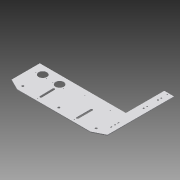
# Autodesk Inventor part: Side-Wall
Saved by Autodesk Inventor 2014 (Build 180170000, 170)
## iProperties
Created: 2013-09-08
Part Number: Side-Wall
Material: Generic
Document SubType Name: Sheet Metal
Designer: hensgen3
Density: 1 g/cm^3
Sheet Metal Rule: Default
Appearance: Aluminum - Polished
Author: hensgen3
Autodesk Inventor part; units mm, degrees
ref_plane "YZ Plane" through (0, 0, 0) normal (1, 0, 0) x (0, 1, 0)
ref_plane "XZ Plane" through (0, 0, 0) normal (0, 1, 0) x (-1, 0, 0)
ref_plane "XY Plane" through (0, 0, 0) normal (0, 0, 1) x (1, 0, 0)
sketch "Sketch1" plane through (0, 0, 0) normal (0, 1, 0) x (-1, 0, 0)
  line L0 (-236.5637, 132.8889) -> (195.2363, 132.8889)
  line L1 (195.2363, 132.8889) -> (195.2363, -19.5111)
  line L2 (195.2363, -19.5111) -> (-236.5637, -19.5111)
  line L3 (-236.5637, -19.5111) -> (-236.5637, 132.8889)
  point P0 (0, 0)
  dimension "d0" = 431.8
  dimension "d2" = 152.4
  measures "d0" distance of L0.start L0.end
  measures "d2" distance of L2.end L0.start
extrude "Plate1" add sketch "Sketch1" along normal blind 3.175
sketch "Sketch2" plane through (0, 3.175, 0) normal (0, 1, 0) x (1, 0, 0)
  line L0 (-195.2363, -132.8889) -> (-195.2363, 19.5111) projected
  line L1 (236.5637, -132.8889) -> (-195.2363, -132.8889) projected
  line L2 (236.5637, 19.5111) -> (236.5637, -132.8889) projected
  line L3 (-195.2363, 19.5111) -> (236.5637, 19.5111) projected
  circle A0 centre (-144.4363, -107.4889) radius 50.8
  line L4 (20.6637, -132.8889) -> (20.6637, -82.0889)
  line L5 (185.7637, -132.8889) -> (185.7637, -82.0889)
  line L6 (-144.4363, -107.4889) -> (-144.4363, -132.8889)
  line L7 (-144.4363, -107.4889) -> (-195.2363, -107.4889)
  line L8 (20.6637, -107.4889) -> (20.6637, -110.6639)
  circle A1 centre (20.6637, -110.6639) radius 50.8
  circle A2 centre (185.7637, -107.4889) radius 50.8
  circle A3 centre (-144.4363, -107.4889) radius 4.7625
  line L9 (-144.4363, -56.6889) -> (185.7637, -56.6889)
  line L10 (-144.4363, -158.2889) -> (185.7637, -158.2889)
  circle A4 centre (20.6637, -110.6639) radius 4.7625
  circle A5 centre (185.7637, -107.4889) radius 4.7625
  point P0 (0, 0)
  dimension "d13" = 50.8
  dimension "d14" = 25.4
  dimension "d15" = 50.8
  dimension "d16" = 3.175
  dimension "d17" = 101.6
  dimension "d18" = 101.6
  dimension "d19" = 9.525
  dimension "d20" = 50.8
  dimension "d21" = 9.525
  dimension "d22" = 9.525
  constraints: 14 end point, 6 centre point, 5 point on circle, 4 coincident, 4 point on line, 3 midpoint, 3 perpendicular, 2 tangent, 1 parallel
  measures "d13" distance of L6.start L7.end
  measures "d14" distance of L6.start L6.end
  measures "d15" distance of L0.start L6.end
  measures "d16" distance of L8.start L8.end
  measures "d17" diameter of A1
  measures "d18" diameter of A2
  measures "d19" diameter of A3
  measures "d20" distance from line of L2 L5.end
  measures "d21" diameter of A4
  measures "d22" diameter of A5
extrude "Cut1" cut sketch "Sketch2" against normal blind 3.175 contours A3 L6 L7 | L7 L6 A3 | L4 A4 | L4 A4 | A5 L5 | L5 A5
sketch "Sketch3" plane through (0, 3.175, 0) normal (0, 1, 0) x (1, 0, 0)
  circle A0 centre (-144.4363, -107.4889) radius 4.7625 projected
  circle A1 centre (20.6637, -110.6639) radius 4.7625 projected
  circle A2 centre (185.7637, -107.4889) radius 4.7625 projected
  line L0 (-195.2363, -132.8889) -> (-195.2363, 19.5111) projected
  line L1 (236.5637, -132.8889) -> (-195.2363, -132.8889) projected
  line L2 (236.5637, 19.5111) -> (236.5637, -132.8889) projected
  circle A3 centre (-144.4363, -107.4889) radius 50.8
  circle A4 centre (20.6637, -110.6639) radius 50.8
  circle A5 centre (185.7637, -107.4889) radius 50.8
  line L3 (-195.2363, -107.4889) -> (-144.4363, -132.8889)
  line L4 (236.5637, -107.4889) -> (185.7637, -132.8889)
  point P0 (0, 0)
  dimension "d25" = 101.6
  dimension "d27" = 101.6
  dimension "d26" = 101.6
  dimension "d31" = 50.8
  dimension "d32" = 50.8
  constraints: 4 end point, 4 point on line, 3 coincident, 2 horizontal alignment, 1 centre point, 4 other
  measures "d26" diameter of A4
  measures "d31" horizontal distance of L3.start L3.end
  measures "d32" horizontal distance of L4.start L4.end
extrude "Cut2" cut sketch "Sketch3" against normal blind 3.175 contours L0 A3 L1 | L3 L1 A3 | L1 A5 L2 | L1 L4 A5 picked at (-178.0457, -118.896) picked at (219.3731, -118.896)
sketch "Sketch4" plane through (0, 3.175, 0) normal (0, 1, 0) x (1, 0, 0)
  line L0 (185.7637, -132.8889) -> (236.5637, -107.4889) projected
  line L1 (236.5637, 19.5111) -> (236.5637, -107.4889) projected
  line L2 (-195.2363, 19.5111) -> (236.5637, 19.5111) projected
  line L3 (-195.2363, -107.4889) -> (-195.2363, 19.5111) projected
  line L4 (-195.2363, -107.4889) -> (-144.4363, -132.8889) projected
  line L5 (185.7637, -132.8889) -> (-144.4363, -132.8889) projected
  circle A0 centre (185.7637, -107.4889) radius 4.7625 projected
  circle A1 centre (20.6637, -110.6639) radius 4.7625 projected
  circle A2 centre (-144.4363, -107.4889) radius 4.7625 projected
  circle A3 centre (-144.4363, -107.4889) radius 50.8
  circle A4 centre (20.6637, -110.6639) radius 50.8
  circle A5 centre (185.7637, -107.4889) radius 50.8
  point P0 (0, 0)
  dimension "d35" = 101.6
  dimension "d36" = 101.6
  dimension "d37" = 101.6
  constraints: 3 centre point, 3 coincident
  measures "d35" diameter of A3
  measures "d36" diameter of A4
  measures "d37" diameter of A5
sketch "Sketch5" plane through (0, 3.175, 0) normal (0, 1, 0) x (1, 0, 0)
  line L0 (185.7637, -132.8889) -> (236.5637, -107.4889) projected
  line L1 (236.5637, 19.5111) -> (236.5637, -107.4889) projected
  line L2 (-195.2363, 19.5111) -> (236.5637, 19.5111) projected
  line L3 (-195.2363, -107.4889) -> (-195.2363, 19.5111) projected
  line L4 (-195.2363, -107.4889) -> (-144.4363, -132.8889) projected
  line L5 (185.7637, -132.8889) -> (-144.4363, -132.8889) projected
  circle A0 centre (185.7637, -107.4889) radius 4.7625 projected
  circle A1 centre (20.6637, -110.6639) radius 4.7625 projected
  circle A2 centre (-144.4363, -107.4889) radius 4.7625 projected
  point P0 (0, 0)
sketch "Sketch6" plane through (0, 3.175, 0) normal (0, 1, 0) x (1, 0, 0)
  line L0 (-195.2363, 19.5111) -> (236.5637, 19.5111) projected
  circle A0 centre (-144.4363, -107.4889) radius 4.7625 projected
  line L1 (-144.4363, -107.4889) -> (-144.4363, 19.5111)
  circle A1 centre (-144.4363, -17.9889) radius 37.5
  circle A2 centre (-68.2363, -17.9889) radius 19.05
  circle A3 centre (-144.4363, -17.9889) radius 18.7706
  circle A4 centre (-68.2363, -17.9889) radius 18.7706
  point P0 (0, 0)
  dimension "d39" = 75
  dimension "d40" = 38.1
  dimension "d41" = 76.2
  dimension "d42" = 37.5412
  dimension "d43" = 37.5412
  constraints: 4 centre point, 2 end point, 2 point on line, 1 coincident, 1 perpendicular, 1 tangent
  measures "d39" diameter of A1
  measures "d40" diameter of A2
  measures "d41" distance of A2.centre A1.centre
  measures "d42" diameter of A3
  measures "d43" diameter of A4
extrude "Cut3" cut sketch "Sketch6" against normal blind 3.175 contours A3 L1 | L1 A3 | A4
sketch "Sketch7" plane through (0, 3.175, 0) normal (0, 1, 0) x (1, 0, 0)
  arc A0 (-36.2323, -12.4614) -> (-39.4073, -9.2864) centre (-39.4073, -12.4614) ccw
  line L0 (-39.4073, -9.2864) -> (-42.3918, -9.2864)
  line L1 (-42.3918, -9.2864) -> (-42.3918, -15.2554)
  line L2 (-42.3918, -15.2554) -> (-49.6689, -15.2554)
  arc A1 (-86.8037, -15.2554) -> (-49.6689, -15.2554) centre (-68.2363, -17.9889) ccw
  line L3 (-86.8037, -15.2554) -> (-94.0808, -15.2554)
  line L4 (-94.0808, -15.2554) -> (-94.0808, -9.2864)
  line L5 (-94.0808, -9.2864) -> (-97.0653, -9.2864)
  arc A2 (-97.0653, -9.2864) -> (-100.2403, -12.4614) centre (-97.0653, -12.4614) ccw
  line L6 (-100.2403, -12.4614) -> (-100.2403, -37.963)
  arc A3 (-100.2403, -37.963) -> (-97.0653, -41.138) centre (-97.0653, -37.963) ccw
  line L7 (-97.0653, -41.138) -> (-39.4073, -41.138)
  arc A4 (-39.4073, -41.138) -> (-36.2323, -37.963) centre (-39.4073, -37.963) ccw
  line L8 (-36.2323, -37.963) -> (-36.2323, -12.4614)
  circle A5 centre (-92.0615, -25.1995) radius 1.8288
  circle A6 centre (-44.4111, -25.1995) radius 1.8288
  line L9 (-118.5918, -15.2554) -> (-125.8689, -15.2554)
  arc A7 (-163.0037, -15.2554) -> (-125.8689, -15.2554) centre (-144.4363, -17.9889) ccw
  line L10 (-163.0037, -15.2554) -> (-170.2808, -15.2554)
  line L11 (-176.4403, -12.4614) -> (-176.4403, -37.963)
  arc A8 (-176.4403, -37.963) -> (-173.2653, -41.138) centre (-173.2653, -37.963) ccw
  line L12 (-173.2653, -41.138) -> (-115.6073, -41.138)
  arc A9 (-115.6073, -41.138) -> (-112.4323, -37.963) centre (-115.6073, -37.963) ccw
  line L13 (-112.4323, -37.963) -> (-112.4323, -12.4614)
  circle A10 centre (-168.2615, -25.1995) radius 1.8288
  circle A11 centre (-120.6111, -25.1995) radius 1.8288
  point P0 (0, 0)
  point P1 (-76.4728, -16.1701)
  point P2 (-115.6073, -12.4614)
  point P3 (-173.2653, -12.4614)
  point P4 (-152.6728, -16.1701)
  constraints: 28 end point, 16 point on circle, 12 centre point
extrude "Cut4" cut sketch "Sketch7" against normal blind 3.175 contours A5 | A6 | A10 | A11
sketch "Sketch8" plane through (0, 3.175, 0) normal (0, 1, 0) x (1, 0, 0)
  line L0 (-195.2363, 19.5111) -> (236.5637, 19.5111) projected
  circle A0 centre (185.7637, -107.4889) radius 4.7625 projected
  circle A1 centre (20.6637, -110.6639) radius 4.7625 projected
  circle A2 centre (-144.4363, -107.4889) radius 4.7625 projected
  line L1 (20.6637, -110.6639) -> (185.7637, -107.4889)
  line L2 (-144.4363, -107.4889) -> (20.6637, -110.6639)
  line L3 (-61.8863, -109.0764) -> (-63.1075, -45.5764)
  line L4 (103.2137, -109.0764) -> (103.2137, -45.5764)
  circle A3 centre (-63.0159, -50.3381) radius 4.7625
  circle A4 centre (-61.8863, -109.0764) radius 4.7625
  line L5 (-58.2613, -50.6132) -> (-57.1247, -109.168)
  line L6 (-66.6479, -108.9849) -> (-67.7775, -50.4299)
  line L7 (20.6637, -110.6639) -> (20.6637, 19.5111)
  circle A5 centre (103.2137, -45.5764) radius 4.7625
  circle A6 centre (103.2137, -109.0764) radius 4.7625
  line L8 (98.4521, -109.168) -> (98.4512, -45.5765)
  line L9 (-57.1247, -109.168) -> (-58.2613, -50.6132)
  line L10 (107.9753, -108.9849) -> (107.9762, -45.5765)
  line L11 (185.7637, -132.8889) -> (-144.4363, -132.8889) projected
  line L12 (-61.8863, -113.8389) -> (-61.8863, -132.8889)
  circle A7 centre (-61.8863, -123.3639) radius 1.8288
  line L13 (103.2137, -113.8389) -> (103.2137, -132.8889)
  circle A8 centre (103.2137, -123.3639) radius 1.8288
  point P0 (0, 0)
  dimension "d48" = 63.5
  dimension "d51" = 63.5
  dimension "d52" = 9.525
  dimension "d53" = 9.525
  dimension "d54" = 9.525
  dimension "d55" = 9.525
  dimension "d65" = 3.6576
  dimension "d66" = 3.6576
  constraints: 24 end point, 11 point on circle, 7 point on line, 6 centre point, 5 midpoint, 4 perpendicular, 3 coincident, 3 tangent, 1 collinear, 1 equal length
  measures "d48" vertical distance of L3.start L3.end
  measures "d51" distance of L4.start L4.end
  measures "d52" diameter of A3
  measures "d53" diameter of A4
  measures "d54" diameter of A5
  measures "d55" diameter of A6
  measures "d65" diameter of A7
  measures "d66" diameter of A8
extrude "Cut5" cut sketch "Sketch8" against normal blind 3.175 contours A6 L4 L1 | L1 A6 | L8 A5 L4 A6 | A4 L2 | L2 L3 A4 L5 | L4 A6 L1 | L4 A5 L10 A6 | A5 | L2 A4 L3 | A4 L3 A3 L5 | A8 L13 | L13 A8 | L6 A3 L3 A4 | A7 L12 | L12 A7 | A3 L3 | A3 L3
sketch "Sketch9" plane through (0, 3.175, 0) normal (0, 1, 0) x (1, 0, 0)
  line L0 (236.5637, 192.7391) -> (236.5637, -107.4889)
  line L1 (192.7868, 192.7391) -> (236.5637, 192.7391)
  line L2 (192.7868, -107.4889) -> (192.7868, 192.7391)
  line L3 (236.5637, -107.4889) -> (192.7868, -107.4889)
  circle A0 centre (214.6752, 78.0581) radius 3.4544
  line L4 (216.7263, -66.2965) -> (216.7263, -70.6018)
  arc A1 (212.6242, -70.6018) -> (216.7263, -70.6018) centre (214.6752, -70.6018) ccw
  line L5 (212.6242, -70.6018) -> (212.6242, -66.2965)
  arc A2 (216.7263, -66.2965) -> (212.6242, -66.2965) centre (214.6752, -66.2965) ccw
  circle A3 centre (214.6752, 93.1203) radius 2.9464
  circle A4 centre (214.6752, 184.5031) radius 2.4575
  circle A5 centre (214.6752, 157.2743) radius 2.94
  circle A6 centre (214.6752, -51.1009) radius 2.9464
  circle A7 centre (214.6752, 142.2248) radius 3.448
  arc A8 (216.7263, -33.9242) -> (212.6242, -33.9242) centre (214.6752, -33.9242) ccw
  line L6 (216.7263, -33.9242) -> (216.7263, -38.2295)
  arc A9 (212.6242, -38.2295) -> (216.7263, -38.2295) centre (214.6752, -38.2295) ccw
  line L7 (212.6242, -38.2295) -> (212.6242, -33.9242)
  point P0 (0, 0)
  point P1 (223.6482, 148.8262)
  constraints: 16 end point, 10 centre point, 8 point on circle
extrude "Cut6" cut sketch "Sketch9" against normal blind 3.175 contours L4 A1 L5 A2 | A6 | L6 A9 L7 A8
sheet face with bend "Face2" sketch "Sketch9" thickness 3.175 toward (0, -1, 0) bend radius 3.175 relief straight relief width 3.175 relief depth 1.5875
bend "Bend1"
hole "Hole1" at (33.3637, 3.175, 5.8889) direction (0, -1, 0) diameter 3.6576 end through all
hole "Hole2" at (147.6637, 3.175, 5.8889) direction (0, -1, 0) diameter 3.6576 end through all
equation "\"d23\" = Thickness"
equation "\"d33\" = Thickness"
equation "\"d44\" = Thickness"
equation "\"d46\" = Thickness"
equation "\"d56\" = Thickness"
equation "\"d58\" = Thickness"
equation "\"d74\" = Thickness"
equation "\"d83\" = Thickness"
equation "\"d60\" = BendRadius"
equation "\"d61\" = BendReliefWidth"
equation "\"d63\" = MinimumRemnant"
equation "\"d62\" = BendReliefDepth"
equation "\"d64\" = BendRadius"
equation "\"BendRadius\" = Thickness"
equation "\"BendReliefWidth\" = Thickness"
equation "\"BendReliefDepth\" = 0.5 * Thickness"
equation "\"CornerReliefSize\" = 4 * Thickness"
equation "\"MinimumRemnant\" = 2 * Thickness"
equation "\"TransitionRadius\" = BendRadius"
equation "\"JacobiRadiusSize\" = BendRadius"
equation "\"GapSize\" = Thickness"
equation "\"d3\" = BendRadius"
equation "\"Thickness\" = 3.175"
body "Solid1"
